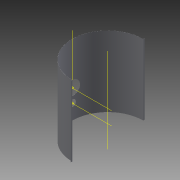
# Autodesk Inventor part: Upper Back Half
Saved by Autodesk Inventor 2015 (Build 190159000, 159)
## iProperties
Created: 2014-06-19
Part Number: Upper Back Half
Material: Generic
Document SubType Name: Modeling
Designer: Aki
Density: 1 g/cm^3
Appearance: Default
Author: Aki
Autodesk Inventor part; units mm, degrees
ref_plane "YZ Plane" through (0, 0, 0) normal (1, 0, 0) x (0, 1, 0)
ref_plane "XZ Plane" through (0, 0, 0) normal (0, 1, 0) x (-1, 0, 0)
sketch "Sketch1" plane through (0, 0, 0) normal (0, 1, 0) x (-1, 0, 0)
  arc A0 (0, -401) -> (0, 401) centre (0, 0) ccw
  line L0 (0, 0) -> (0, 401) construction
  line L1 (0, 0) -> (0, -401) construction
  arc A1 (0, -400) -> (0, 400) centre (0, 0) ccw
  line L2 (0, 0) -> (0, 400) construction
  line L3 (0, 0) -> (0, -400) construction
  line L4 (0, 401) -> (0, 400)
  line L5 (0, -400) -> (0, -401)
  dimension "d0" = 401
  dimension "d1" = 180
  dimension "d2" = 400
  dimension "d3" = 180
  constraints: 12 end point, 4 point on circle, 2 centre point, 2 coincident, 1 collinear
  measures "d0" radius of A0
  measures "d1" angle of L0 L1
  measures "d2" radius of A1
  measures "d3" angle of L2 L3
extrude "Extrusion1" add sketch "Sketch1" along normal blind 796
sketch "Sketch2" plane through (0, 0, 0) normal (0, 1, 0) x (-1, 0, 0)
  line L0 (0, -401) -> (1, -401)
  line L1 (1, -401) -> (1, -416)
  line L2 (1, -416) -> (0, -416)
  line L3 (0, -416) -> (0, -401)
  point P0 (0, 0)
  dimension "d6" = 1
  dimension "d7" = 15
  constraints: 8 end point, 2 parallel, 1 horizontal, 1 perpendicular
  measures "d6" distance of L1.end L2.end
  measures "d7" distance of L0.end L1.end
extrude "Extrusion2" add sketch "Sketch2" along normal blind 796
sketch "Sketch4" plane through (0, 0, 0) normal (0, 1, 0) x (-1, 0, 0)
  line L0 (0, 401) -> (1, 401)
  line L1 (1, 401) -> (1, 416)
  line L2 (1, 416) -> (0, 416)
  line L3 (0, 416) -> (0, 401)
  point P0 (0, 0)
  dimension "d10" = 1
  dimension "d11" = 15
  constraints: 8 end point, 2 parallel, 1 horizontal, 1 perpendicular
  measures "d10" distance of L2.end L1.end
  measures "d11" distance of L1.end L0.end
extrude "Extrusion3" add sketch "Sketch4" along normal blind 796
ref_plane "Work Plane1" through (-401, 0, 0) normal (-1, 0, 0) x (0, -1, 0)
sketch "Sketch6" plane through (-401, 0, 0) normal (-1, 0, 0) x (0, -1, 0)
  circle A0 centre (-168.5, 0) radius 39
  line L0 (-796, 401) -> (-796, -401) projected
  point P0 (0, 0)
  dimension "d15" = 78
  dimension "d16" = 627.5
  constraints: 1 centre point
  measures "d15" diameter of A0
  measures "d16" distance from line of L0 A0.centre
hole "Hole1" at (-401, 168.5, 0) direction (1, 0, 0) diameter 78 end through all
sketch "Sketch7" plane through (-401, 0, 0) normal (-1, 0, 0) x (0, -1, 0)
  circle A0 centre (-317.5, 0) radius 80
  line L0 (-796, 401) -> (-796, -401) projected
  point P0 (0, 0)
  dimension "d26" = 160
  dimension "d27" = 478.5
  constraints: 1 centre point
  measures "d26" diameter of A0
  measures "d27" distance from line of L0 A0.centre
hole "Hole2" at (-401, 317.5, 0) direction (1, 0, 0) diameter 160 end through all
body "Solid1"
